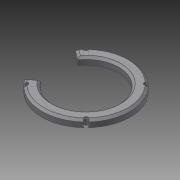
# Autodesk Inventor part: cover
Saved by Autodesk Inventor 2018 (Build 220112000, 112)
## iProperties
Created: 2019-02-21
Part Number: cover
Material: 一般
Document SubType Name: Modeling
Designer: ku_sk
Density: 1 g/cm^3
Appearance: 既定
Author: ku_sk
Autodesk Inventor part; units mm, degrees
ref_plane "YZ Plane" through (0, 0, 0) normal (1, 0, 0) x (0, 1, 0)
ref_plane "XZ Plane" through (0, 0, 0) normal (0, 1, 0) x (-1, 0, 0)
ref_plane "XY Plane" through (0, 0, 0) normal (0, 0, 1) x (1, 0, 0)
sketch "スケッチ1" plane through (0, 0, 0) normal (0, 0, 1) x (1, 0, 0)
  arc A0 (-18.8405, -13.1923) -> (-18.8405, 13.1923) centre (0, 0) ccw
  line L0 (-36.6725, 0) -> (42.2787, 0) projected
  arc A1 (-25.3937, -17.7809) -> (-25.3937, 17.7809) centre (0, 0) ccw
  line L1 (-25.3937, -17.7809) -> (-18.8405, -13.1923)
  line L2 (-18.8405, 13.1923) -> (-25.3937, 17.7809)
  point P0 (23, 0)
  dimension "d0" = 23
  dimension "d1" = 8
  dimension "d2" = 290
  constraints: 5 point on circle, 4 end point, 2 centre point, 2 line through centre, 1 coincident, 1 point on line
  measures "d0" radius of A0
  measures "d1" radial gap between concentric circles of A0 A1
extrude "押し出し1" add sketch "スケッチ1" along normal blind 5
chamfer "面取り1" distance 1.5 angle 45 5 edges at (31, 0, 5) (6.9162, -21.9355, 5) (6.9162, 21.9355, 5) (-22.1171, 15.4866, 5) (-22.1171, -15.4866, 5)
sketch "スケッチ2" plane through (0, 0, 5) normal (0, 0, 1) x (1, 0, 0)
  circle A0 centre (-21.2132, 21.2132) radius 1.5 projected
  circle A1 centre (21.2132, 21.2132) radius 1.5 projected
  circle A2 centre (21.2132, -21.2132) radius 1.5 projected
  circle A3 centre (-21.2132, -21.2132) radius 1.5 projected
  point P0 (0, 0)
extrude "押し出し2" cut sketch "スケッチ2" against normal through all
